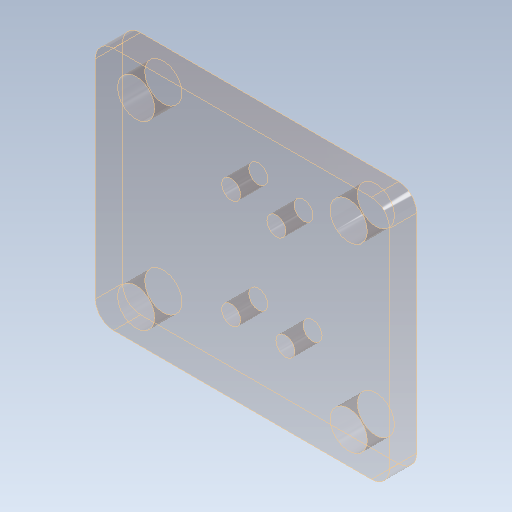
# Autodesk Inventor part: Pump Mounting Plate
Saved by Autodesk Inventor 2021 (Build 250183000, 183)
## iProperties
Created: 2019-11-22
Part Number: Pump Mounting Plate
Material: Generic
Document SubType Name: Modeling
Designer: jgray
Density: 1 g/cm^3
Appearance: Default
Author: jgray
Autodesk Inventor part; units mm, degrees
ref_plane "YZ Plane" through (0, 0, 0) normal (1, 0, 0) x (0, 1, 0)
ref_plane "XZ Plane" through (0, 0, 0) normal (0, 1, 0) x (-1, 0, 0)
ref_plane "XY Plane" through (0, 0, 0) normal (0, 0, 1) x (1, 0, 0)
sketch "Sketch1" plane through (0, 0, 0) normal (0, 0, 1) x (1, 0, 0)
  line L0 (0, 0) -> (12.5, 0) construction
  line L1 (12.5, 0) -> (12.5, 17) construction
  line L2 (12.5, 17) -> (0, 17) construction
  line L3 (0, 17) -> (0, 0) construction
  line L4 (5, 3) -> (11, 3) construction
  line L5 (11, 3) -> (11, 15) construction
  line L6 (11, 15) -> (5, 15) construction
  line L7 (5, 15) -> (5, 3) construction
  line L8 (-10, 22) -> (22.5, 22)
  line L9 (22.5, 22) -> (22.5, -5)
  line L10 (22.5, -5) -> (-10, -5)
  line L11 (-10, -5) -> (-10, 22)
  circle A0 centre (-5.5, 18.5) radius 2.05
  circle A1 centre (-5.5, -1.5) radius 2.05
  circle A2 centre (18, -1.5) radius 2.05
  circle A3 centre (18, 18.5) radius 2.05
  point P0 (10, 14)
  dimension "d0" = 12.5
  dimension "d1" = 17
  dimension "d2" = 6
  dimension "d3" = 12
  dimension "d4" = 5
  dimension "d5" = 2
  dimension "d6" = 1
  dimension "d7" = 1
  dimension "d8" = 32.5
  dimension "d9" = 27
  dimension "d10" = 5
  dimension "d11" = 10
  dimension "d12" = 4.1
  dimension "d13" = 4.1
  dimension "d14" = 4.1
  dimension "d15" = 4.1
  dimension "d16" = 3.5
  dimension "d17" = 3.5
  dimension "d18" = 3.5
  dimension "d19" = 3.5
  dimension "d20" = 4.5
  dimension "d21" = 4.5
  dimension "d22" = 4.5
  dimension "d23" = 4.5
  constraints: 24 end point, 6 parallel, 4 centre point, 3 coincident, 3 horizontal, 3 perpendicular
  measures "d0" distance of L2.end L1.end
  measures "d1" distance of L1.end L0.end
  measures "d2" distance of L6.end L5.end
  measures "d3" distance of L5.end L4.end
  measures "d4" distance between parallel lines of L3 L7
  measures "d5" distance between parallel lines of L2 L6
  measures "d6" distance from line of L5 point (10, 14)
  measures "d7" distance from line of L6 point (10, 14)
  measures "d8" distance of L9.end L10.end
  measures "d9" distance of L8.end L9.end
  measures "d10" distance between parallel lines of L8 L2
  measures "d11" distance between parallel lines of L9 L1
  measures "d12" diameter of A0
  measures "d13" diameter of A1
  measures "d14" diameter of A2
  measures "d15" diameter of A3
  measures "d16" distance from line of L8 A0.centre
  measures "d17" distance from line of L10 A1.centre
  measures "d18" distance from line of L10 A2.centre
  measures "d19" distance from line of L8 A3.centre
  measures "d20" distance from line of L11 A0.centre
  measures "d21" distance from line of L11 A1.centre
  measures "d22" distance from line of L9 A3.centre
  measures "d23" distance from line of L9 A2.centre
extrude "Extrusion1" add sketch "Sketch1" along normal blind 3
hole "Hole1" at (10, 14, 0) at (5, 15, 0) at (5, 3, 0) at (11, 3, 0) direction (0, 0, 1) diameter 2.1 end through all
fillet "Fillet1" radius 2 4 edges at (-10, 22, 1.5) (22.5, 22, 1.5) (22.5, -5, 1.5) (-10, -5, 1.5)
body "Solid1"
